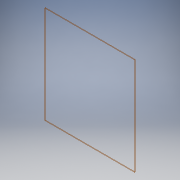
# Autodesk Inventor part: Back Panel
Saved by Autodesk Inventor 2016 (Build 200138000, 138)
## iProperties
Created: 2017-11-01
Part Number: Back Panel
Material: Wood (Cherry)
Document SubType Name: Modeling
Designer: mathaetaes
Density: 0.63 g/cm^3
Appearance: Cherry - Natural Low Gloss
Author: mathaetaes
Autodesk Inventor part; units mm, degrees
ref_plane "YZ Plane" through (0, 0, 0) normal (1, 0, 0) x (0, 1, 0)
ref_plane "XZ Plane" through (0, 0, 0) normal (0, 1, 0) x (-1, 0, 0)
ref_plane "XY Plane" through (0, 0, 0) normal (0, 0, 1) x (1, 0, 0)
sketch "Sketch1" plane through (0, 0, 0) normal (0, 0, 1) x (1, 0, 0)
  line L0 (0, 889) -> (819.15, 889)
  line L1 (819.15, 889) -> (819.15, 0)
  line L2 (819.15, 0) -> (0, 0)
  line L3 (0, 0) -> (0, 889)
  dimension "d0" = 819.15
  dimension "d1" = 889
  constraints: 8 end point, 2 parallel, 1 coincident, 1 horizontal, 1 perpendicular
  measures "d0" distance of L0.start L0.end
  measures "d1" distance of L0.end L1.end
extrude "Board" add sketch "Sketch1" along normal blind 6.35
body "Solid1"
